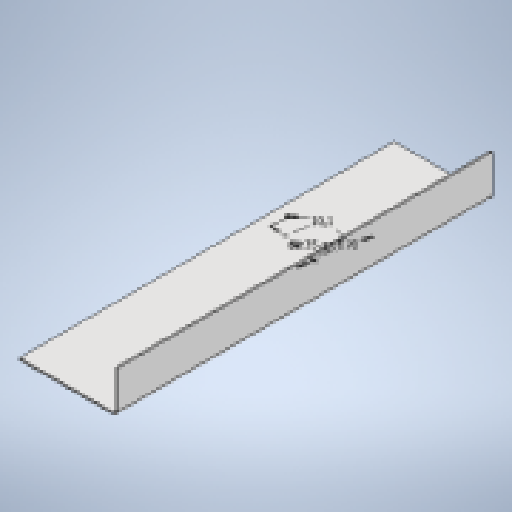
# Autodesk Inventor part: MNT-CDF-603 CAP
Saved by Autodesk Inventor 2025 (Build 290162010, 162A)
## iProperties
Created: 2025-01-16
Part Number: MNT-CDF-603 CAP
Material: Stainless Steel
Document SubType Name: Sheet Metal
Designer: pokla
Density: 8 g/cm^3
Sheet Metal Rule: AISI304 2mm Die16
Appearance: Default
Flat Pattern Width: 14.6202 cm
Flat Pattern Length: 34.7014 cm
Flat Pattern Area: 507.341 cm^2
Sheet Metal Width: 146,202 mm
Sheet Metal Length: 347,014 mm
Sheet Metal Area: 50734,146 mm^2
Author: pokla
Autodesk Inventor part; units mm, degrees
ref_plane "YZ Plane" through (0, 0, 0) normal (1, 0, 0) x (0, 1, 0)
ref_plane "XZ Plane" through (0, 0, 0) normal (0, 1, 0) x (-1, 0, 0)
ref_plane "XY Plane" through (0, 0, 0) normal (0, 0, 1) x (1, 0, 0)
sketch "Sketch1" plane through (0, 0, 0) normal (0, 0, 1) x (1, 0, 0)
  line L0 (-52.5, 168.5) -> (52.5, 168.5)
  line L1 (52.5, 168.5) -> (52.5, -168.5)
  line L2 (52.5, -168.5) -> (-52.5, -168.5)
  line L3 (-52.5, -168.5) -> (-52.5, 168.5)
  line L4 (-52.5, 168.5) -> (52.5, -168.5) construction
  point P0 (0, 0)
  point P1 (0, 0)
  dimension "d0" = 105
  dimension "d1" = 337
  measures "d0" distance of L0.start L0.end
  measures "d1" distance of L2.end L0.start
extrude "Plate1" add sketch "Sketch1" along normal blind 2
sketch "Sketch4" plane through (50.5, 168.5, 0) normal (1, 0, 0) x (0, 1, 0)
  line L0 (-337, 0) -> (0, 0)
  line L1 (0, 0) -> (0, 45)
  line L2 (0, 45) -> (-337, 45)
  line L3 (-337, 45) -> (-337, 0)
  constraints: 6 end point, 1 horizontal, 1 perpendicular, 1 vertical
edge flange "Flange1" height 45 angle 90 thickness 2 bend radius 2.75 thickness toward (1, 0, 0) relief round relief width 2 relief depth 1 edges at (52.5, 0, 2) wall of the first edge with corners at (50.5, -168.5, 0) (50.5, 168.5, 0) (50.5, 168.5, 45) (50.5, -168.5, 45)
bend "Bend1"
corner "Corner1"
sketch "Sketch5" plane through (0, 0, 0) normal (0, 0, -1) x (-1, 0, 0)
  line L0 (-47.75, 168.5) -> (-47.75, -168.5) projected
  line L1 (52.5, -168.5) -> (-47.75, -168.5) projected
  line L2 (52.5, 168.5) -> (52.5, -168.5) projected
  line L3 (-47.75, 168.5) -> (52.5, 168.5) projected
  line L4 (52.5, -168.5) -> (52.5, -179.0367)
  line L5 (-47.75, -168.5) -> (52.5, -168.5) projected
  line L6 (52.5, -179.0367) -> (-47.75, -168.5)
  point P0 (0, 0)
  dimension "d25" = 6
  constraints: 4 end point, 1 vertical
  measures "d25" angle of L1 L6
extrude "Extrusion2" add sketch "Sketch5" against normal up to surface (2 mm away) contours L1 L4 L6
sketch "Sketch6" plane through (0, 0, 0) normal (0, 0, -1) x (-1, 0, 0)
  line L0 (-47.75, 168.5) -> (-47.75, -168.5) construction
  line L1 (-47.75, -168.5) -> (52.5, -179.0367) projected
  line L2 (52.5, 168.5) -> (52.5, -179.0367) projected
  line L3 (-47.75, 168.5) -> (52.5, 168.5) construction
  line L4 (47.5274, -178.5141) -> (52.5, -131.2028)
  line L5 (-47.75, -168.5) -> (52.5, -179.0367) projected
  point P0 (0, 0)
  dimension "d29" = 5
  constraints: 2 end point, 2 point on line, 1 perpendicular
  measures "d29" distance from line of L1.end L4
extrude "Cut1" cut sketch "Sketch6" against normal blind 2
sketch "Sketch7" plane through (0, 0, 0) normal (0, 0, 1) x (1, 0, 0)
  line L0 (47.75, -168.5) -> (-47.5274, -178.5141) projected
  circle A0 centre (42.7027, -144.3955) radius 5.05
  line L1 (42.7027, -144.3955) -> (35.3858, -74.779) construction
  line L2 (33.4146, -127.7754) -> (29.7561, -92.9671)
  circle A1 centre (35.3858, -74.779) radius 5.05
  line L3 (-20.6271, -115.859) -> (42.7027, -144.3955) construction
  line L4 (33.4146, -127.7754) -> (-5.0522, -96.6256) construction
  line L5 (29.7561, -92.9671) -> (-5.0522, -96.6256)
  line L6 (-1.3937, -131.4339) -> (33.4146, -127.7754)
  line L7 (29.7561, -92.9671) -> (-1.3937, -131.4339) construction
  line L8 (-5.0522, -96.6256) -> (-1.3937, -131.4339)
  line L9 (31.5853, -110.3712) -> (-20.6271, -115.859) construction
  line L10 (35.3858, -74.779) -> (-20.6271, -115.859) construction
  circle A2 centre (-20.6271, -115.859) radius 5.05
  point P0 (0, 0)
  point P1 (14.1812, -112.2005)
  dimension "d32" = 35
  dimension "d33" = 35
  dimension "d34" = 10.1
  dimension "d35" = 70
  dimension "d36" = 60
  dimension "d37" = 25
  dimension "d38" = 10
  dimension "d39" = 42
  constraints: 20 end point, 3 centre point, 3 midpoint, 3 parallel, 2 perpendicular, 1 equal radius, 2 other
  measures "d32" distance of L6.start L4.end
  measures "d33" distance of L4.end L2.end
  measures "d34" diameter of A2
  measures "d35" distance of L1.start L1.end
  measures "d36" distance from line of L3.start L1
  measures "d37" distance from line of L1 point (14.181, -112.2)
  measures "d38" distance from line of L0.start L2
  measures "d39" distance between parallel lines of L0 L6
extrude "Extrusion3" cut sketch "Sketch7" along normal through all
equation "\"d30\" = Thickness"
equation "\"d33\" = d32"
equation "\"d2\" = Thickness"
equation "\"d15\" = BendReliefWidth"
equation "\"d16\" = BendReliefDepth"
equation "\"d17\" = MinimumRemnant"
equation "\"d18\" = TransitionRadius"
equation "\"d21\" = BendRadius"
equation "\"d22\" = CornerReliefSize"
equation "\"d23\" = GapSize"
equation "\"d24\" = JacobiRadiusSize"
equation "\"BendReliefWidth\" = Thickness"
equation "\"BendReliefDepth\" = 0.5 * Thickness"
equation "\"CornerReliefSize\" = 4 * Thickness"
equation "\"MinimumRemnant\" = 2 * Thickness"
equation "\"TransitionRadius\" = BendRadius"
equation "\"JacobiRadiusSize\" = BendRadius"
equation "\"GapSize\" = Thickness"
equation "\"Thickness\" = 2"
equation "\"BendRadius\" = 2.75"
body "Solid1"
